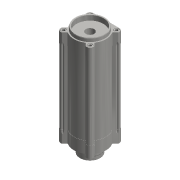
# Autodesk Inventor part: ESBF-BS-100-100---(ZR_-_-)
Saved by Autodesk Inventor 2021 (Build 250183000, 183)
## iProperties
Part Number: ESBF-BS-100-100---(ZR_-_-)
Material: Steel AISI 1080
Catalog Web Link: www.cadenas.de
Description: ESBF-(ZR)-Electro-cylinder
Vendor: FESTO
Document SubType Name: Modeling
Designer: partserver
Manufacturer: FESTO
Mass: 16884 g
Surface Area: 3014.64 cm^2
Volume: 2150.83 cm^3
Density: 7.85 g/cm^3
Appearance: Steel
Category: PARTsolutions
Company: FESTO
PSOL_IDENT_0: {$CADENAS_DATA\23d-libs\festo\parts\e\esbf\parts\esbf_zr.prj},210 {VTYP=3D},{NB=ESBF-BS-100-100---(Z
PSOL_IDENT_1: R_-_-)},{LINA=ESBF-BS-100-100---(ZR_-_-)},{NN=ESBF-(ZR)},{DATE=27.05.2021 13:20:18},{GEOMDATE=27.05.
PSOL_IDENT_2: 2021 13:19:59},{VERSION=},{LINEID=30},{WBVAR=HUB,SCEL,BWE},{WBNUMERIC=HUB}  {NB=ESBF-BS-100-100---(Z
PSOL_IDENT_3: R_-_-)},{LINA=ESBF-BS-100-100---(ZR_-_-)},{KT=DUMMY},{TNR=574092},{TYP=ESBF-BS-100},{KDM=100},{HUB=1
PSOL_IDENT_4: 00},{SCEL=-},{BWE=-},{A=29.000},{ANG=45.000},{B=70.000},{B1=68.000},{BE1=18.000},{BG=17.000},{D1=50.
PSOL_IDENT_5: 000},{D2=24.000},{D2R=15.000},{D3=100.000},{D3R=15.800},{D5=90.000},{E=110.000},{E1=0.000},{EG=20.50
PSOL_IDENT_6: 0},{G=39.000},{G1=39.000},{HE=4.000},{R1=10.500},{R1I=10.000},{R2=107.600},{TG=89.000},{RI=53.250},{
PSOL_IDENT_7: RK=1.500},{T5=16.500},{J2=0.000},{L10=21.000},{L14=30.000},{L16=20.200},{L18=0.000},{L1=33.000},{L2=
PSOL_IDENT_8: 224.000},{L3=39.500},{L7=68.500},{M1=10.000},{PL=0.000},{SW3=6.000},{SWT=25.900},{VA=12.000},{VD=20.
PSOL_IDENT_9: 000},{D100=0.000},{GUA=28.000},{B2=5.000},{D6=51.500},{D7=61.200},{BWE1='-','F1A'}
NB: ESBF-BS-100-100---(ZR_-_-)
NN: ESBF-(ZR)
NT: Electro-cylinder
NBSYN: $TYP.-$HUB.---(ZR_$SCEL._$BWE.)
LINA: ESBF-BS-100-100---(ZR_-_-)
CATALOG: Festo
TNR: 574092
TYP: ESBF-BS-100
KDM: 100
HUB: 100
SCEL: -
BWE: -
A: 29
ANG: 45
B: 70
B1: 68
BE1: 18
BG: 17
D1: 50
D2: 24
D2R: 15
D3: 100
D3R: 15.8
D5: 90
E: 110
E1: 0
EG: 20.5
G: 39
G1: 39
HE: 4
R1: 10.5
R1I: 10
R2: 107.6
TG: 89
RI: 53.25
RK: 1.5
T5: 16.5
J2: 0
L10: 21
L14: 30
L16: 20.2
L18: 0
L1: 33
L2: 224
L3: 39.5
L7: 68.5
M1: 10
PL: 0
SW3: 6
SWT: 25.9
VA: 12
VD: 20
D100: 0
GUA: 28
B2: 5
D6: 51.5
D7: 61.2
SUPPLIER: FESTO
ARTICLENO: ESBF-BS-100-100---(ZR_-_-)
BOMINFO: ESBF-BS-100-100---(ZR_-_-)
CREATOR: CADENAS GmbH
Title: ESBF-BS-100-100---(ZR_-_-)
Author: Cadenas PARTsolutions
Comments: Electro-cylinder
Autodesk Inventor part; units mm, degrees
sketch "Sketch_1" plane through (0, 0, -39) normal (0, 0, 1) x (1, 0, 0)
  arc A0 (-55, 40.7721) -> (-54.5607, 39.7114) centre (-53.5, 40.7721) ccw
  line L0 (-54.5607, 39.7114) -> (-45.5959, 30.7466)
  arc A1 (-45.391, 28.8808) -> (-45.5959, 30.7466) centre (-46.6565, 29.686) ccw
  arc A2 (-45.391, 28.8808) -> (-45.391, -28.8808) centre (0, 0) ccw
  arc A3 (-45.5959, -30.7466) -> (-45.391, -28.8808) centre (-46.6565, -29.686) ccw
  line L1 (-45.5959, -30.7466) -> (-54.5607, -39.7114)
  arc A4 (-54.5607, -39.7114) -> (-55, -40.7721) centre (-53.5, -40.7721) ccw
  line L2 (-55, -40.7721) -> (-55, -44.5)
  arc A5 (-55, -44.5) -> (-44.5, -55) centre (-44.5, -44.5) ccw
  line L3 (-44.5, -55) -> (-40.7721, -55)
  arc A6 (-40.7721, -55) -> (-39.7114, -54.5607) centre (-40.7721, -53.5) ccw
  line L4 (-39.7114, -54.5607) -> (-30.7466, -45.5959)
  arc A7 (-28.8808, -45.391) -> (-30.7466, -45.5959) centre (-29.686, -46.6565) ccw
  arc A8 (-28.8808, -45.391) -> (28.8808, -45.391) centre (0, 0) ccw
  arc A9 (30.7466, -45.5959) -> (28.8808, -45.391) centre (29.686, -46.6565) ccw
  line L5 (30.7466, -45.5959) -> (39.7114, -54.5607)
  arc A10 (39.7114, -54.5607) -> (40.7721, -55) centre (40.7721, -53.5) ccw
  line L6 (40.7721, -55) -> (44.5, -55)
  arc A11 (44.5, -55) -> (55, -44.5) centre (44.5, -44.5) ccw
  line L7 (55, -44.5) -> (55, -40.7721)
  arc A12 (55, -40.7721) -> (54.5607, -39.7114) centre (53.5, -40.7721) ccw
  line L8 (54.5607, -39.7114) -> (45.5959, -30.7466)
  arc A13 (45.391, -28.8808) -> (45.5959, -30.7466) centre (46.6565, -29.686) ccw
  arc A14 (45.391, -28.8808) -> (45.391, 28.8808) centre (0, 0) ccw
  arc A15 (45.5959, 30.7466) -> (45.391, 28.8808) centre (46.6565, 29.686) ccw
  line L9 (45.5959, 30.7466) -> (54.5607, 39.7114)
  arc A16 (54.5607, 39.7114) -> (55, 40.7721) centre (53.5, 40.7721) ccw
  line L10 (55, 40.7721) -> (55, 44.5)
  arc A17 (55, 44.5) -> (44.5, 55) centre (44.5, 44.5) ccw
  line L11 (44.5, 55) -> (-44.5, 55)
  arc A18 (-44.5, 55) -> (-55, 44.5) centre (-44.5, 44.5) ccw
  line L12 (-55, 44.5) -> (-55, 40.7721)
  constraints: 38 point on circle, 26 end point, 19 centre point
extrude "Extrusion1" add sketch "Sketch_1" along normal blind 39
sketch "Sketch_8" plane through (0, 0, -39) normal (0, 0, 1) x (1, 0, 0)
  line L0 (-50, 73) -> (50, 73)
  line L1 (-41.5, 68.75) -> (-41.5, 55)
  line L2 (-41.5, 55) -> (-39.2483, 51.1)
  arc A0 (-39.2483, 51.1) -> (-39.0751, 51) centre (-39.0751, 51.2) ccw
  line L3 (-39.0751, 51) -> (-38.3734, 51)
  arc A1 (-38.3734, 51) -> (-38.232, 51.0586) centre (-38.3734, 51.2) ccw
  line L4 (-38.232, 51.0586) -> (-34.2906, 55)
  line L5 (-34.2906, 55) -> (34.2906, 55)
  line L6 (34.2906, 55) -> (38.232, 51.0586)
  arc A2 (38.232, 51.0586) -> (38.3734, 51) centre (38.3734, 51.2) ccw
  line L7 (38.3734, 51) -> (39.0751, 51)
  arc A3 (39.0751, 51) -> (39.2483, 51.1) centre (39.0751, 51.2) ccw
  line L8 (39.2483, 51.1) -> (41.5, 55)
  line L9 (41.5, 55) -> (41.5, 68.75)
  line L10 (41.5, 68.75) -> (-41.5, 68.75)
  constraints: 22 end point, 8 point on circle, 4 centre point
revolve "Revolution1" cut sketch "Sketch_8" angle 360 about axis through (-50, 73, -39) along (-1, 0, 0)
sketch "Sketch_21" plane through (0, 0, -39) normal (0, 0, 1) x (1, 0, 0)
  line L0 (50, -74) -> (-50, -74)
  line L1 (-41.5, -68.75) -> (41.5, -68.75)
  line L2 (41.5, -68.75) -> (41.5, -55)
  line L3 (41.5, -55) -> (39.2483, -51.1)
  arc A0 (39.2483, -51.1) -> (39.0751, -51) centre (39.0751, -51.2) ccw
  line L4 (39.0751, -51) -> (25.0048, -51)
  arc A1 (-25.0048, -51) -> (25.0048, -51) centre (0, 0) ccw
  line L5 (-25.0048, -51) -> (-39.0751, -51)
  arc A2 (-39.0751, -51) -> (-39.2483, -51.1) centre (-39.0751, -51.2) ccw
  line L6 (-39.2483, -51.1) -> (-41.5, -55)
  line L7 (-41.5, -55) -> (-41.5, -68.75)
  constraints: 16 end point, 6 point on circle, 3 centre point
revolve "Revolution2" cut sketch "Sketch_21" angle 360 about axis through (50, -74, -39) along (1, 0, 0)
sketch "Sketch_23" plane through (0, 0, -39) normal (0, 0, 1) x (1, 0, 0)
  line L0 (74, 50) -> (74, -50)
  line L1 (51, -25.0048) -> (51, -39.0751)
  arc A0 (51, -39.0751) -> (51.1, -39.2483) centre (51.2, -39.0751) ccw
  line L2 (51.1, -39.2483) -> (55, -41.5)
  line L3 (55, -41.5) -> (68.75, -41.5)
  line L4 (68.75, -41.5) -> (68.75, 41.5)
  line L5 (68.75, 41.5) -> (55, 41.5)
  line L6 (55, 41.5) -> (51.1, 39.2483)
  arc A1 (51.1, 39.2483) -> (51, 39.0751) centre (51.2, 39.0751) ccw
  line L7 (51, 39.0751) -> (51, 25.0048)
  arc A2 (51, -25.0048) -> (51, 25.0048) centre (0, 0) ccw
  constraints: 16 end point, 6 point on circle, 3 centre point
revolve "Revolution3" cut sketch "Sketch_23" angle 360 about axis through (74, 50, -39) along (0, 1, 0)
sketch "Sketch_24" plane through (0, 0, -39) normal (0, 0, 1) x (1, 0, 0)
  line L0 (-74, -50) -> (-74, 50)
  line L1 (-68.75, -41.5) -> (-55, -41.5)
  line L2 (-55, -41.5) -> (-51.1, -39.2483)
  arc A0 (-51.1, -39.2483) -> (-51, -39.0751) centre (-51.2, -39.0751) ccw
  line L3 (-51, -39.0751) -> (-51, -25.0048)
  arc A1 (-51, 25.0048) -> (-51, -25.0048) centre (0, 0) ccw
  line L4 (-51, 25.0048) -> (-51, 39.0751)
  arc A2 (-51, 39.0751) -> (-51.1, 39.2483) centre (-51.2, 39.0751) ccw
  line L5 (-51.1, 39.2483) -> (-55, 41.5)
  line L6 (-55, 41.5) -> (-68.75, 41.5)
  line L7 (-68.75, 41.5) -> (-68.75, -41.5)
  constraints: 16 end point, 6 point on circle, 3 centre point
revolve "Revolution4" cut sketch "Sketch_24" angle 360 about axis through (-74, -50, -39) along (0, -1, 0)
sketch "Sketch_41" plane through (0, 0, 0) normal (1, 0, 0) x (0, 1, 0)
  line L0 (0, -285) -> (0, -39)
  line L1 (0, -39) -> (5, -39)
  line L2 (5, -39) -> (5, -285)
  line L3 (5, -285) -> (0, -285)
  line L4 (0, -285) -> (0, -39)
  constraints: 10 end point
revolve "Revolution5" add sketch "Sketch_41" angle 360 about axis through (0, 0, -285) along (0, 0, -1)
sketch "Sketch_5" plane through (0, 0, -285) normal (0, 0, 1) x (1, 0, 0)
  arc A0 (-55, 40.7721) -> (-54.5607, 39.7114) centre (-53.5, 40.7721) ccw
  line L0 (-54.5607, 39.7114) -> (-45.5959, 30.7466)
  arc A1 (-45.391, 28.8808) -> (-45.5959, 30.7466) centre (-46.6565, 29.686) ccw
  arc A2 (-45.391, 28.8808) -> (-45.391, -28.8808) centre (0, 0) ccw
  arc A3 (-45.5959, -30.7466) -> (-45.391, -28.8808) centre (-46.6565, -29.686) ccw
  line L1 (-45.5959, -30.7466) -> (-54.5607, -39.7114)
  arc A4 (-54.5607, -39.7114) -> (-55, -40.7721) centre (-53.5, -40.7721) ccw
  line L2 (-55, -40.7721) -> (-55, -44.5)
  arc A5 (-55, -44.5) -> (-44.5, -55) centre (-44.5, -44.5) ccw
  line L3 (-44.5, -55) -> (-40.7721, -55)
  arc A6 (-40.7721, -55) -> (-39.7114, -54.5607) centre (-40.7721, -53.5) ccw
  line L4 (-39.7114, -54.5607) -> (-30.7466, -45.5959)
  arc A7 (-28.8808, -45.391) -> (-30.7466, -45.5959) centre (-29.686, -46.6565) ccw
  arc A8 (-28.8808, -45.391) -> (28.8808, -45.391) centre (0, 0) ccw
  arc A9 (30.7466, -45.5959) -> (28.8808, -45.391) centre (29.686, -46.6565) ccw
  line L5 (30.7466, -45.5959) -> (39.7114, -54.5607)
  arc A10 (39.7114, -54.5607) -> (40.7721, -55) centre (40.7721, -53.5) ccw
  line L6 (40.7721, -55) -> (44.5, -55)
  arc A11 (44.5, -55) -> (55, -44.5) centre (44.5, -44.5) ccw
  line L7 (55, -44.5) -> (55, -40.7721)
  arc A12 (55, -40.7721) -> (54.5607, -39.7114) centre (53.5, -40.7721) ccw
  line L8 (54.5607, -39.7114) -> (45.5959, -30.7466)
  arc A13 (45.391, -28.8808) -> (45.5959, -30.7466) centre (46.6565, -29.686) ccw
  arc A14 (45.391, -28.8808) -> (45.391, 28.8808) centre (0, 0) ccw
  arc A15 (45.5959, 30.7466) -> (45.391, 28.8808) centre (46.6565, 29.686) ccw
  line L9 (45.5959, 30.7466) -> (54.5607, 39.7114)
  arc A16 (54.5607, 39.7114) -> (55, 40.7721) centre (53.5, 40.7721) ccw
  line L10 (55, 40.7721) -> (55, 44.5)
  arc A17 (55, 44.5) -> (44.5, 55) centre (44.5, 44.5) ccw
  line L11 (44.5, 55) -> (-44.5, 55)
  arc A18 (-44.5, 55) -> (-55, 44.5) centre (-44.5, 44.5) ccw
  line L12 (-55, 44.5) -> (-55, 40.7721)
  constraints: 38 point on circle, 26 end point, 19 centre point
extrude "Extrusion2" add sketch "Sketch_5" against normal blind 39
sketch "Sketch_4" plane through (0, 0, -285) normal (0, 0, 1) x (1, 0, 0)
  line L0 (-50, 74) -> (50, 74)
  line L1 (-41.5, 68.75) -> (-41.5, 55)
  line L2 (-41.5, 55) -> (-39.2483, 51.1)
  arc A0 (-39.2483, 51.1) -> (-39.0751, 51) centre (-39.0751, 51.2) ccw
  line L3 (-39.0751, 51) -> (-38.3734, 51)
  arc A1 (-38.3734, 51) -> (-38.232, 51.0586) centre (-38.3734, 51.2) ccw
  line L4 (-38.232, 51.0586) -> (-34.2906, 55)
  line L5 (-34.2906, 55) -> (34.2906, 55)
  line L6 (34.2906, 55) -> (38.232, 51.0586)
  arc A2 (38.232, 51.0586) -> (38.3734, 51) centre (38.3734, 51.2) ccw
  line L7 (38.3734, 51) -> (39.0751, 51)
  arc A3 (39.0751, 51) -> (39.2483, 51.1) centre (39.0751, 51.2) ccw
  line L8 (39.2483, 51.1) -> (41.5, 55)
  line L9 (41.5, 55) -> (41.5, 68.75)
  line L10 (41.5, 68.75) -> (-41.5, 68.75)
  constraints: 22 end point, 8 point on circle, 4 centre point
revolve "Revolution6" cut sketch "Sketch_4" angle 360 about axis through (-50, 74, -285) along (-1, 0, 0)
sketch "Sketch_25" plane through (0, 0, -285) normal (0, 0, 1) x (1, 0, 0)
  line L0 (50, -74) -> (-50, -74)
  line L1 (-41.5, -73.3333) -> (41.5, -73.3333)
  line L2 (41.5, -73.3333) -> (41.5, -55)
  line L3 (41.5, -55) -> (39.2483, -51.1)
  arc A0 (39.2483, -51.1) -> (39.0751, -51) centre (39.0751, -51.2) ccw
  line L4 (39.0751, -51) -> (25.0048, -51)
  arc A1 (-25.0048, -51) -> (25.0048, -51) centre (0, 0) ccw
  line L5 (-25.0048, -51) -> (-39.0751, -51)
  arc A2 (-39.0751, -51) -> (-39.2483, -51.1) centre (-39.0751, -51.2) ccw
  line L6 (-39.2483, -51.1) -> (-41.5, -55)
  line L7 (-41.5, -55) -> (-41.5, -73.3333)
  constraints: 16 end point, 6 point on circle, 3 centre point
revolve "Revolution7" cut sketch "Sketch_25" angle 360 about axis through (50, -74, -285) along (1, 0, 0)
sketch "Sketch_26" plane through (0, 0, -285) normal (0, 0, 1) x (1, 0, 0)
  line L0 (74, 50) -> (74, -50)
  line L1 (51, -25.0048) -> (51, -39.0751)
  arc A0 (51, -39.0751) -> (51.1, -39.2483) centre (51.2, -39.0751) ccw
  line L2 (51.1, -39.2483) -> (55, -41.5)
  line L3 (55, -41.5) -> (68.75, -41.5)
  line L4 (68.75, -41.5) -> (68.75, 41.5)
  line L5 (68.75, 41.5) -> (55, 41.5)
  line L6 (55, 41.5) -> (51.1, 39.2483)
  arc A1 (51.1, 39.2483) -> (51, 39.0751) centre (51.2, 39.0751) ccw
  line L7 (51, 39.0751) -> (51, 25.0048)
  arc A2 (51, -25.0048) -> (51, 25.0048) centre (0, 0) ccw
  constraints: 16 end point, 6 point on circle, 3 centre point
revolve "Revolution8" cut sketch "Sketch_26" angle 360 about axis through (74, 50, -285) along (0, 1, 0)
sketch "Sketch_27" plane through (0, 0, -285) normal (0, 0, 1) x (1, 0, 0)
  line L0 (-74, -50) -> (-74, 50)
  line L1 (-68.75, -41.5) -> (-55, -41.5)
  line L2 (-55, -41.5) -> (-51.1, -39.2483)
  arc A0 (-51.1, -39.2483) -> (-51, -39.0751) centre (-51.2, -39.0751) ccw
  line L3 (-51, -39.0751) -> (-51, -25.0048)
  arc A1 (-51, 25.0048) -> (-51, -25.0048) centre (0, 0) ccw
  line L4 (-51, 25.0048) -> (-51, 39.0751)
  arc A2 (-51, 39.0751) -> (-51.1, 39.2483) centre (-51.2, 39.0751) ccw
  line L5 (-51.1, 39.2483) -> (-55, 41.5)
  line L6 (-55, 41.5) -> (-68.75, 41.5)
  line L7 (-68.75, 41.5) -> (-68.75, -41.5)
  constraints: 16 end point, 6 point on circle, 3 centre point
revolve "Revolution9" cut sketch "Sketch_27" angle 360 about axis through (-74, -50, -285) along (0, -1, 0)
sketch "Sketch_43" plane through (0, 0, -39) normal (0, 0, 1) x (1, 0, 0)
  arc A0 (-54.3387, -41.9115) -> (-41.9115, -54.3387) centre (-44.75, -44.75) ccw
  arc A1 (-41.9115, -54.3387) -> (-41.6786, -54.1551) centre (-42.025, -53.9551) ccw
  line L0 (-41.6786, -54.1551) -> (-39.8281, -50.95)
  arc A2 (-39.4817, -50.75) -> (-39.8281, -50.95) centre (-39.4817, -51.15) ccw
  line L1 (-39.4817, -50.75) -> (-36.42, -50.75)
  arc A3 (-36.42, -50.75) -> (-36.1372, -50.6328) centre (-36.42, -50.35) ccw
  line L2 (-36.1372, -50.6328) -> (-30.5642, -45.0599)
  arc A4 (-28.6952, -44.857) -> (-30.5642, -45.0599) centre (-29.5035, -46.1205) ccw
  arc A5 (-28.6952, -44.857) -> (28.6952, -44.857) centre (0, 0) ccw
  arc A6 (30.5642, -45.0599) -> (28.6952, -44.857) centre (29.5035, -46.1205) ccw
  line L3 (30.5642, -45.0599) -> (36.1372, -50.6328)
  arc A7 (36.1372, -50.6328) -> (36.42, -50.75) centre (36.42, -50.35) ccw
  line L4 (36.42, -50.75) -> (39.4817, -50.75)
  arc A8 (39.8281, -50.95) -> (39.4817, -50.75) centre (39.4817, -51.15) ccw
  line L5 (39.8281, -50.95) -> (41.6786, -54.1551)
  arc A9 (41.6786, -54.1551) -> (41.9115, -54.3387) centre (42.025, -53.9551) ccw
  arc A10 (41.9115, -54.3387) -> (54.3387, -41.9115) centre (44.75, -44.75) ccw
  arc A11 (54.3387, -41.9115) -> (54.1551, -41.6786) centre (53.9551, -42.025) ccw
  line L6 (54.1551, -41.6786) -> (50.95, -39.8281)
  arc A12 (50.75, -39.4817) -> (50.95, -39.8281) centre (51.15, -39.4817) ccw
  line L7 (50.75, -39.4817) -> (50.75, -36.42)
  arc A13 (50.75, -36.42) -> (50.6328, -36.1372) centre (50.35, -36.42) ccw
  line L8 (50.6328, -36.1372) -> (45.0599, -30.5642)
  arc A14 (44.857, -28.6952) -> (45.0599, -30.5642) centre (46.1205, -29.5035) ccw
  arc A15 (44.857, -28.6952) -> (44.1971, 29.7014) centre (0, 0) ccw
  line L9 (44.1971, 29.7014) -> (50.6328, 36.1372)
  arc A16 (50.6328, 36.1372) -> (50.75, 36.42) centre (50.35, 36.42) ccw
  line L10 (50.75, 36.42) -> (50.75, 39.4817)
  arc A17 (50.95, 39.8281) -> (50.75, 39.4817) centre (51.15, 39.4817) ccw
  line L11 (50.95, 39.8281) -> (54.1551, 41.6786)
  arc A18 (54.1551, 41.6786) -> (54.3387, 41.9115) centre (53.9551, 42.025) ccw
  arc A19 (54.3387, 41.9115) -> (41.9115, 54.3387) centre (44.75, 44.75) ccw
  arc A20 (41.9115, 54.3387) -> (41.6786, 54.1551) centre (42.025, 53.9551) ccw
  line L12 (41.6786, 54.1551) -> (39.8281, 50.95)
  arc A21 (39.4817, 50.75) -> (39.8281, 50.95) centre (39.4817, 51.15) ccw
  line L13 (39.4817, 50.75) -> (38.8713, 50.75)
  arc A22 (37.8107, 51.1893) -> (38.8713, 50.75) centre (38.8713, 52.25) ccw
  line L14 (37.8107, 51.1893) -> (34.25, 54.75)
  line L15 (34.25, 54.75) -> (-34.25, 54.75)
  line L16 (-34.25, 54.75) -> (-37.8107, 51.1893)
  arc A23 (-38.8713, 50.75) -> (-37.8107, 51.1893) centre (-38.8713, 52.25) ccw
  line L17 (-38.8713, 50.75) -> (-39.4817, 50.75)
  arc A24 (-39.8281, 50.95) -> (-39.4817, 50.75) centre (-39.4817, 51.15) ccw
  line L18 (-39.8281, 50.95) -> (-41.6786, 54.1551)
  arc A25 (-41.6786, 54.1551) -> (-41.9115, 54.3387) centre (-42.025, 53.9551) ccw
  arc A26 (-41.9115, 54.3387) -> (-54.3387, 41.9115) centre (-44.75, 44.75) ccw
  arc A27 (-54.3387, 41.9115) -> (-54.1551, 41.6786) centre (-53.9551, 42.025) ccw
  line L19 (-54.1551, 41.6786) -> (-50.95, 39.8281)
  arc A28 (-50.75, 39.4817) -> (-50.95, 39.8281) centre (-51.15, 39.4817) ccw
  line L20 (-50.75, 39.4817) -> (-50.75, 36.42)
  arc A29 (-50.75, 36.42) -> (-50.6328, 36.1372) centre (-50.35, 36.42) ccw
  line L21 (-50.6328, 36.1372) -> (-44.1971, 29.7014)
  arc A30 (-44.1971, 29.7014) -> (-44.857, -28.6952) centre (0, 0) ccw
  arc A31 (-45.0599, -30.5642) -> (-44.857, -28.6952) centre (-46.1205, -29.5035) ccw
  line L22 (-45.0599, -30.5642) -> (-50.6328, -36.1372)
  arc A32 (-50.6328, -36.1372) -> (-50.75, -36.42) centre (-50.35, -36.42) ccw
  line L23 (-50.75, -36.42) -> (-50.75, -39.4817)
  arc A33 (-50.95, -39.8281) -> (-50.75, -39.4817) centre (-51.15, -39.4817) ccw
  line L24 (-50.95, -39.8281) -> (-54.1551, -41.6786)
  arc A34 (-54.1551, -41.6786) -> (-54.3387, -41.9115) centre (-53.9551, -42.025) ccw
  constraints: 70 point on circle, 50 end point, 35 centre point
extrude "Extrusion3" add sketch "Sketch_43" against normal blind 246
sketch "Sketch_3" plane through (0, 0, 0) normal (1, 0, 0) x (0, 1, 0)
  line L0 (0, 0) -> (0, 38)
  line L1 (0, 38) -> (25.75, 38)
  arc A0 (25.75, 38) -> (26.6564, 36.3255) centre (27.75, 38) ccw
  line L2 (26.6564, 36.3255) -> (30.6, 33.75)
  line L3 (30.6, 33.75) -> (30.6, 33)
  line L4 (30.6, 33) -> (33.5, 33)
  line L5 (33.5, 33) -> (34, 32.5)
  line L6 (34, 32.5) -> (34, 21.7321)
  line L7 (34, 21.7321) -> (35, 20)
  line L8 (35, 20) -> (35, 0)
  line L9 (35, 0) -> (0, 0)
  line L10 (0, 0) -> (0, 38)
  constraints: 22 end point, 2 point on circle, 1 centre point
revolve "Revolution10" add sketch "Sketch_3" angle 360 about axis through (0, 0, 0) along (0, 0, -1)
sketch "Sketch_45" plane through (0, 0, -255.5) normal (0, 0, 1) x (1, 0, 0)
  line L0 (0, 54.45) -> (0, 54.75)
  line L1 (0, 54.75) -> (7.05, 54.75)
  line L2 (7.05, 54.75) -> (7.05, 54.45)
  line L3 (7.05, 54.45) -> (0, 54.45)
  line L4 (0, 54.45) -> (0, 54.75)
  constraints: 10 end point
revolve "Revolution11" cut sketch "Sketch_45" angle 360 about axis through (0, 54.45, -255.5) along (0, -1, 0)
sketch "Sketch_9" plane through (44.5, 0, 0) normal (1, 0, 0) x (0, 0, -1)
  line L0 (30, 44.5) -> (0, 44.5)
  line L1 (0, 44.5) -> (0, 52.4)
  line L2 (0, 52.4) -> (30, 52.4)
  line L3 (30, 52.4) -> (30, 44.5)
  line L4 (30, 44.5) -> (0, 44.5)
  constraints: 10 end point
revolve "Revolution12" cut sketch "Sketch_9" angle 360 about axis through (44.5, 44.5, -30) along (0, 0, -1)
pattern_linear "Rectangular Pattern1" count 2 spacing 89 along (-1, 0, 0) count 2 spacing 89 along (0, -1, 0) of "Revolution12"
sketch "Sketch_11" plane through (44.5, 0, 0) normal (1, 0, 0) x (0, 0, -1)
  line L0 (30, 44.5) -> (0, 44.5)
  line L1 (0, 44.5) -> (0, 51)
  line L2 (0, 51) -> (1, 52)
  line L3 (1, 52) -> (30, 52)
  line L4 (30, 52) -> (30, 44.5)
  line L5 (30, 44.5) -> (0, 44.5)
  constraints: 12 end point
revolve "Revolution13" add sketch "Sketch_11" angle 360 about axis through (44.5, 44.5, -30) along (0, 0, -1)
pattern_linear "Rectangular Pattern2" count 2 spacing 89 along (-1, 0, 0) count 2 spacing 89 along (0, -1, 0) of "Revolution13"
sketch "Sketch_17" plane through (44.5, 0, 0) normal (1, 0, 0) x (0, 0, -1)
  line L0 (22.2577, 44.5) -> (0, 44.5)
  line L1 (0, 44.5) -> (0, 49.5)
  line L2 (0, 49.5) -> (0.812, 48.688)
  line L3 (0.812, 48.688) -> (20.2, 48.688)
  line L4 (20.2, 48.688) -> (22.2577, 47.5)
  line L5 (22.2577, 47.5) -> (22.2577, 44.5)
  line L6 (22.2577, 44.5) -> (0, 44.5)
  constraints: 14 end point
revolve "Revolution14" cut sketch "Sketch_17" angle 360 about axis through (44.5, 44.5, -22.2577) along (0, 0, -1)
thread "Thread1" size "M10x1.5" class "6H" standard "ISO Metric profile" length 16.188
sketch "Sketch_18" plane through (0, 0, 0) normal (0, 0, 1) x (1, 0, 0)
  line L0 (41.5, 42.7679) -> (44.5, 41.0359)
  line L1 (44.5, 41.0359) -> (47.5, 42.7679)
  line L2 (47.5, 42.7679) -> (47.5, 46.2321)
  line L3 (47.5, 46.2321) -> (44.5, 47.9641)
  line L4 (44.5, 47.9641) -> (41.5, 46.2321)
  line L5 (41.5, 46.2321) -> (41.5, 42.7679)
  constraints: 12 end point
extrude "Extrusion4" cut sketch "Sketch_18" against normal blind 25.9
pattern_linear "Rectangular Pattern3" count 2 spacing 89 along (-1, 0, 0) count 2 spacing 89 along (0, -1, 0) of "Revolution14"
pattern_linear "Rectangular Pattern4" count 2 spacing 89 along (-1, 0, 0) count 2 spacing 89 along (0, -1, 0) of "Extrusion4"
sketch "Sketch_22" plane through (0, 0, 0) normal (1, 0, 0) x (0, 1, 0)
  line L0 (0, -336) -> (0, -324)
  line L1 (0, -324) -> (50, -324)
  line L2 (50, -324) -> (50, -334)
  line L3 (50, -334) -> (49.2721, -336)
  line L4 (49.2721, -336) -> (0, -336)
  line L5 (0, -336) -> (0, -324)
  constraints: 12 end point
revolve "Revolution15" add sketch "Sketch_22" angle 360 about axis through (0, 0, -336) along (0, 0, -1)
sketch "Sketch_2" plane through (0, 0, 0) normal (1, 0, 0) x (0, 1, 0)
  line L0 (0, -336) -> (0, -285)
  line L1 (0, -285) -> (14, -285)
  line L2 (14, -285) -> (14, -319.5)
  line L3 (14, -319.5) -> (45, -319.5)
  line L4 (45, -319.5) -> (45, -335)
  line L5 (45, -335) -> (45.364, -336)
  line L6 (45.364, -336) -> (0, -336)
  line L7 (0, -336) -> (0, -285)
  constraints: 16 end point
revolve "Revolution16" cut sketch "Sketch_2" angle 360 about axis through (0, 0, -336) along (0, 0, -1)
sketch "Sketch21" plane through (0, 0, -324) normal (0, 0, -1) x (-1, 0, 0)
  point P0 (-44.5, 44.5)
hole "Hole1" at (44.5, 44.5, -324) direction (0, 0, 1) diameter 15.8 depth 30
pattern_linear "Rectangular Pattern5" count 2 spacing 89 along (-1, 0, 0) count 2 spacing 89 along (0, -1, 0) of "Hole1"
sketch "Sketch_30" plane through (44.5, 0, 0) normal (1, 0, 0) x (0, 0, -1)
  line L0 (324, 44.5) -> (294, 44.5)
  line L1 (294, 44.5) -> (294, 52)
  line L2 (294, 52) -> (323, 52)
  line L3 (323, 52) -> (324, 51)
  line L4 (324, 51) -> (324, 44.5)
  line L5 (324, 44.5) -> (294, 44.5)
  constraints: 12 end point
revolve "Revolution17" add sketch "Sketch_30" angle 360 about axis through (44.5, 44.5, -324) along (0, 0, -1)
pattern_linear "Rectangular Pattern6" count 2 spacing 89 along (-1, 0, 0) count 2 spacing 89 along (0, -1, 0) of "Revolution17"
sketch "Sketch_36" plane through (44.5, 0, 0) normal (1, 0, 0) x (0, 0, -1)
  line L0 (324, 44.5) -> (301.7423, 44.5)
  line L1 (301.7423, 44.5) -> (301.7423, 47.5)
  line L2 (301.7423, 47.5) -> (303.8, 48.688)
  line L3 (303.8, 48.688) -> (323.188, 48.688)
  line L4 (323.188, 48.688) -> (324, 49.5)
  line L5 (324, 49.5) -> (324, 44.5)
  line L6 (324, 44.5) -> (301.7423, 44.5)
  constraints: 14 end point
revolve "Revolution18" cut sketch "Sketch_36" angle 360 about axis through (44.5, 44.5, -324) along (0, 0, -1)
thread "Thread2" size "M10x1.5" class "6H" standard "ISO Metric profile" length 16.188
pattern_linear "Rectangular Pattern7" count 2 spacing 89 along (-1, 0, 0) count 2 spacing 89 along (0, -1, 0) of "Revolution18"
sketch "Sketch_38" plane through (0, 0, -324) normal (0, 0, 1) x (1, 0, 0)
  line L0 (41.5, 42.7679) -> (44.5, 41.0359)
  line L1 (44.5, 41.0359) -> (47.5, 42.7679)
  line L2 (47.5, 42.7679) -> (47.5, 46.2321)
  line L3 (47.5, 46.2321) -> (44.5, 47.9641)
  line L4 (44.5, 47.9641) -> (41.5, 46.2321)
  line L5 (41.5, 46.2321) -> (41.5, 42.7679)
  constraints: 12 end point
extrude "Extrusion5" cut sketch "Sketch_38" along normal blind 25.9
pattern_linear "Rectangular Pattern8" count 2 spacing 89 along (-1, 0, 0) count 2 spacing 89 along (0, -1, 0) of "Extrusion5"
sketch "Sketch25" plane through (0, 0, -285) normal (0, 0, -1) x (-1, 0, 0)
  point P0 (0, 0)
hole "Hole2" at (0, 0, -285) direction (0, 0, 1) diameter 50 depth 323 counterbore diameter 100 counterbore depth 133.3333
ref_plane "GUA_XY" through (0, 0, -319.5) normal (0, 0, 1) x (0, 1, 0)
ref_plane "GUA_YZ" through (0, 0, -319.5) normal (0, 1, 0) x (-1, 0, 0)
ref_plane "GUA_ZX" through (0, 0, -319.5) normal (-1, 0, 0) x (0, 0, 1)
ref_plane "KS_XY" through (0, 0, -285) normal (0, 0, 1) x (1, 0, 0)
ref_plane "KS_YZ" through (0, 0, -285) normal (1, 0, 0) x (0, 1, 0)
ref_plane "KS_ZX" through (0, 0, -285) normal (0, 1, 0) x (0, 0, 1)
ref_plane "KSA_XY" through (0, 0, -285) normal (0, 0, -1) x (1, 0, 0)
ref_plane "KSA_YZ" through (0, 0, -285) normal (1, 0, 0) x (0, -1, 0)
ref_plane "KSA_ZX" through (0, 0, -285) normal (0, -1, 0) x (0, 0, -1)
ref_plane "PLUG_XY" through (0, 54.75, -255.5) normal (0, -1, 0) x (1, 0, 0)
ref_plane "PLUG_YZ" through (0, 54.75, -255.5) normal (1, 0, 0) x (0, 0, 1)
ref_plane "PLUG_ZX" through (0, 54.75, -255.5) normal (0, 0, 1) x (0, -1, 0)
ref_plane "SENSOR_XY" through (0, 55, -162) normal (0, 0, 1) x (1, 0, 0)
ref_plane "SENSOR_YZ" through (0, 55, -162) normal (1, 0, 0) x (0, 1, 0)
ref_plane "SENSOR_ZX" through (0, 55, -162) normal (0, 1, 0) x (0, 0, 1)
ref_plane "START_XY" through (0, 0, 0) normal (0, 0, -1) x (1, 0, 0)
ref_plane "START_YZ" through (0, 0, 0) normal (1, 0, 0) x (0, -1, 0)
ref_plane "START_ZX" through (0, 0, 0) normal (0, -1, 0) x (0, 0, -1)
body "Solid1"
